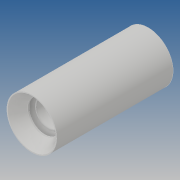
# Autodesk Inventor part: cartridge_locker
Saved by Autodesk Inventor 2019 (Build 230136000, 136)
## iProperties
Created: 2019-03-09
Part Number: cartridge_locker
Material: Générique
Document SubType Name: Modeling
Designer: Theo
Density: 1 g/cm^3
Appearance: Par défaut
Author: Theo
Autodesk Inventor part; units mm, degrees
ref_plane "XZ Plane" through (0, 0, 0) normal (0, 1, 0) x (-1, 0, 0)
ref_plane "XY Plane" through (0, 0, 0) normal (0, 0, 1) x (1, 0, 0)
sketch "Esquisse1" plane through (0, 0, 0) normal (1, 0, 0) x (0, 1, 0)
  line L0 (9.5, 0) -> (9.5, -10)
  line L1 (0, 0) -> (0, -29.8331)
  line L2 (9.5, 0) -> (15, 0)
  line L3 (9.5, -10) -> (7.5, -10)
  line L4 (7.5, -10) -> (7.5, -15)
  line L5 (7.5, -15) -> (12, -25)
  line L6 (12, -25) -> (12, -70)
  line L7 (15, -70) -> (12, -70)
  line L8 (15, -70) -> (15, 0)
  dimension "d0" = 19
  dimension "d2" = 10
  dimension "d3" = 2
  dimension "d4" = 5
  dimension "d6" = 10
  dimension "d7" = 70
  dimension "d16" = 3
  dimension "d19" = 30
  constraints: 18 end point, 5 vertical, 3 horizontal, 1 horizontal alignment
  measures "d0" diameter of L0 L1
  measures "d2" distance of L0.start L0.end
  measures "d3" distance of L0.end L3.end
  measures "d4" distance of L3.end L4.end
  measures "d6" vertical distance of L4.end L5.end
  measures "d7" distance from line of L2 L7.start
  measures "d16" distance between parallel lines of L8 L6
  measures "d19" diameter of L8 L1
revolve "Révolution1" add sketch "Esquisse1" angle 360 about axis through (0, 0, 0) along (0, 0, -1)
chamfer "Chanfrein1" distance 5 distance2 7 1 edges at (0, -9.5, 0) measured on face at (-1.9544, 12.9294, 0)
chamfer "Chanfrein2" distance 2 angle 45 1 edges at (0, -12, -70)
ref_plane "Plan de construction1" through (-15, 0, -35) normal (1, 0, 0) x (0, 1, 0)
sketch "Esquisse3" plane through (-15, 0, -35) normal (1, 0, 0) x (0, 1, 0)
  circle A0 centre (0, 30) radius 3
  point P0 (0, 35)
  dimension "d23" = 6
  dimension "d24" = 5
  constraints: 1 centre point, 1 vertical alignment
  measures "d23" diameter of A0
  measures "d24" distance of point (0, 35) A0.centre
extrude "Extrusion1" [suppressed]
sketch "Esquisse4" plane through (0, 0, 0) normal (1, 0, 0) x (0, 1, 0)
  line L0 (-15, 0) -> (15, 0) projected
  line L1 (-15, -70) -> (15, -70) projected
  line L2 (-9.5, -10) -> (-9.5, -7) projected
  line L3 (-9.5, -10) -> (9.5, -10) projected
  line L4 (-7.5, -15) -> (-7.5, -10) projected
  line L5 (-14.5, 0) -> (-9.5, -7) projected
  line L6 (-9.5, -7.9) -> (-11.8748, -8.7815)
  line L7 (-11.8748, -8.7815) -> (-9.5199, -12.0265)
  line L8 (-9.5199, -12.0265) -> (-8, -10)
  circle A0 centre (-9.5, -9.5) radius 1.5 construction
  line L9 (0, -72) -> (0, 12) projected
  point P0 (0, 0)
  dimension "d32" = 3
  dimension "d37" = 0.5
  dimension "d38" = 1.5
  dimension "d39" = 2.1
  constraints: 6 end point, 3 point on line, 3 tangent, 1 centre point, 1 equal length
  measures "d32" diameter of A0
  measures "d37" distance of L2.start A0.centre
  measures "d38" distance of L8.end L2.start
  measures "d39" distance of L2.start L6.start
revolve "Révolution2" cut sketch "Esquisse4" angle 360 about axis through (0, 0, -10) along (0, 0, 1) contours L2 L3 L8 L7 L6
